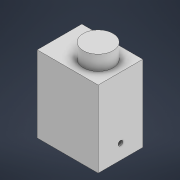
# Autodesk Inventor part: SolidnoidV
Saved by Autodesk Inventor 2022 (Build 260153070, 153G)
## iProperties
Created: 2021-07-21
Part Number: SolidnoidV
Material: Generic
Document SubType Name: Modeling
Designer: Eakawit_kor
Density: 1 g/cm^3
Appearance: Default
Author: Eakawit_kor
Autodesk Inventor part; units mm, degrees
ref_plane "YZ Plane" through (0, 0, 0) normal (1, 0, 0) x (0, 1, 0)
ref_plane "XZ Plane" through (0, 0, 0) normal (0, 1, 0) x (-1, 0, 0)
ref_plane "XY Plane" through (0, 0, 0) normal (0, 0, 1) x (1, 0, 0)
sketch "Sketch1" plane through (0, 0, 0) normal (0, 0, 1) x (1, 0, 0)
  line L0 (0, 0) -> (41, 0)
  line L1 (41, 0) -> (41, 61.3)
  line L2 (41, 61.3) -> (0, 61.3)
  line L3 (0, 61.3) -> (0, 0)
  dimension "d0" = 61.3
  dimension "d1" = 41
  constraints: 8 end point, 2 parallel, 1 horizontal, 1 perpendicular
  measures "d0" distance of L2.end L0.start
  measures "d1" distance of L0.start L0.end
extrude "Extrusion1" add sketch "Sketch1" along normal blind 30
sketch "Sketch2" plane through (0, 0, 0) normal (-1, 0, 0) x (0, 0, 1)
  circle A0 centre (15, 10) radius 1.5875
  line L0 (0, 0) -> (30, 0) projected
  line L1 (0, 61.3) -> (0, 0) projected
  dimension "d4" = 3.175
  dimension "d5" = 10
  dimension "d6" = 15
  constraints: 1 centre point
  measures "d4" diameter of A0
  measures "d5" distance from line of L0 A0.centre
  measures "d6" distance from line of L1 A0.centre
extrude "Extrusion2" cut sketch "Sketch2" against normal through all
sketch "Sketch3" plane through (0, 61.3, 0) normal (0, 1, 0) x (1, 0, 0)
  line L0 (0, 0) -> (0, -30) projected
  line L1 (41, 0) -> (41, -30) projected
  line L2 (0, 0) -> (41, 0)
  line L3 (41, 0) -> (41, -30)
  line L4 (41, -30) -> (0, -30)
  line L5 (0, -30) -> (0, 0)
  circle A0 centre (26, -15) radius 10
  dimension "d9" = 15
  dimension "d10" = 15
  dimension "d11" = 20
  constraints: 8 end point, 2 parallel, 1 centre point, 1 horizontal, 1 perpendicular
  measures "d9" distance from line of L2 A0.centre
  measures "d10" distance from line of L1 A0.centre
  measures "d11" diameter of A0
extrude "Extrusion3" cut sketch "Sketch3" against normal blind 10
body "Solid1"
